Autodesk Fusion 360 part; units mm, degrees
(part 2 of 2)
  spline S19 degree 5 poles (10.4079, -1.3878) (10.4039, -1.3845) (10.3958, -1.3779) (10.3838, -1.3681) (10.3676, -1.3551) (10.3475, -1.3389) (10.3272, -1.3228) (10.3069, -1.3069) (10.2866, -1.2911) (10.2663, -1.2755) (10.2458, -1.2599) (10.2254, -1.2445) (10.2049, -1.2292) (10.1844, -1.214) (10.1638, -1.199) (10.1432, -1.1841) (10.1225, -1.1693) (10.1018, -1.1547) (10.0811, -1.1402) (10.0603, -1.1258) (10.0395, -1.1116) (10.0186, -1.0975) (9.9977, -1.0835) (9.9768, -1.0697) (9.9558, -1.056) (9.9348, -1.0424) (9.9137, -1.029) (9.8926, -1.0157) (9.8715, -1.0026) (9.8503, -0.9896) (9.8291, -0.9768) (9.8078, -0.9641) (9.7866, -0.9516) (9.7652, -0.9392) (9.7439, -0.9269) (9.7225, -0.9149) (9.7011, -0.9029) (9.6796, -0.8911) (9.6581, -0.8795) (9.6366, -0.8681) (9.615, -0.8568) (9.5934, -0.8456) (9.5717, -0.8347) (9.5501, -0.8239) (9.5283, -0.8132) (9.5066, -0.8028) (9.4848, -0.7925) (9.463, -0.7824) (9.4412, -0.7724) (9.4193, -0.7627) (9.3974, -0.7531) (9.3754, -0.7438) (9.3534, -0.7346) (9.3314, -0.7257) (9.3094, -0.7169) (9.2873, -0.7084) (9.2652, -0.7) (9.2431, -0.6918) (9.2209, -0.6839) (9.1987, -0.6761) (9.1764, -0.6686) (9.1542, -0.6615) (9.1318, -0.6547) (9.1095, -0.6482) (9.0871, -0.6419) (9.0646, -0.636) (9.0422, -0.6301) (9.0197, -0.6245) (8.9973, -0.619) (8.9748, -0.6141) (8.9522, -0.6098) (8.934, -0.6071) (8.9203, -0.6056) (8.9112, -0.6048) (8.9066, -0.6045) knots -1 -1 -1 -1 -1 -1 -0.98571429 -0.97142857 -0.95714286 -0.94285714 -0.92857143 -0.91428571 -0.9 -0.88571429 -0.87142857 -0.85714286 -0.84285714 -0.82857143 -0.81428571 -0.8 -0.78571429 -0.77142857 -0.75714286 -0.74285714 -0.72857143 -0.71428571 -0.7 -0.68571429 -0.67142857 -0.65714286 -0.64285714 -0.62857143 -0.61428571 -0.6 -0.58571429 -0.57142857 -0.55714286 -0.54285714 -0.52857143 -0.51428571 -0.5 -0.48571429 -0.47142857 -0.45714286 -0.44285714 -0.42857143 -0.41428571 -0.4 -0.38571429 -0.37142857 -0.35714286 -0.34285714 -0.32857143 -0.31428571 -0.3 -0.28571429 -0.27142857 -0.25714286 -0.24285714 -0.22857143 -0.21428571 -0.2 -0.18571429 -0.17142857 -0.15714286 -0.14285714 -0.12857143 -0.11428571 -0.1 -0.08571429 -0.07142857 -0.05714286 -0.04285714 -0.02857143 -0.01428571 0 0 0 0 0 0
  line L19 (8.9066, -0.6045) -> (8.2303, -0.5577)
  arc A20 (8.2303, -0.5577) -> (8.2303, 0.5577) centre (0, 0) ccw
  line L20 (8.2303, 0.5577) -> (8.9066, 0.6045)
  spline S20 degree 5 poles (8.9066, 0.6045) (8.9112, 0.6048) (8.9203, 0.6056) (8.934, 0.6071) (8.9522, 0.6098) (8.9748, 0.6141) (8.9973, 0.619) (9.0197, 0.6245) (9.0422, 0.6301) (9.0646, 0.636) (9.0871, 0.6419) (9.1095, 0.6482) (9.1318, 0.6547) (9.1542, 0.6615) (9.1764, 0.6686) (9.1987, 0.6761) (9.2209, 0.6839) (9.2431, 0.6918) (9.2652, 0.7) (9.2873, 0.7084) (9.3094, 0.7169) (9.3314, 0.7257) (9.3534, 0.7346) (9.3754, 0.7438) (9.3974, 0.7531) (9.4193, 0.7627) (9.4412, 0.7724) (9.463, 0.7824) (9.4848, 0.7925) (9.5066, 0.8028) (9.5283, 0.8132) (9.5501, 0.8239) (9.5717, 0.8347) (9.5934, 0.8456) (9.615, 0.8568) (9.6366, 0.8681) (9.6581, 0.8795) (9.6796, 0.8911) (9.7011, 0.9029) (9.7225, 0.9149) (9.7439, 0.9269) (9.7652, 0.9392) (9.7866, 0.9516) (9.8078, 0.9641) (9.8291, 0.9768) (9.8503, 0.9896) (9.8715, 1.0026) (9.8926, 1.0157) (9.9137, 1.029) (9.9348, 1.0424) (9.9558, 1.056) (9.9768, 1.0697) (9.9977, 1.0835) (10.0186, 1.0975) (10.0395, 1.1116) (10.0603, 1.1258) (10.0811, 1.1402) (10.1018, 1.1547) (10.1225, 1.1693) (10.1432, 1.1841) (10.1638, 1.199) (10.1844, 1.214) (10.2049, 1.2292) (10.2254, 1.2445) (10.2458, 1.2599) (10.2663, 1.2755) (10.2866, 1.2911) (10.3069, 1.3069) (10.3272, 1.3228) (10.3475, 1.3389) (10.3676, 1.3551) (10.3838, 1.3681) (10.3958, 1.3779) (10.4039, 1.3845) (10.4079, 1.3878) knots 0 0 0 0 0 0 0.01428571 0.02857143 0.04285714 0.05714286 0.07142857 0.08571429 0.1 0.11428571 0.12857143 0.14285714 0.15714286 0.17142857 0.18571429 0.2 0.21428571 0.22857143 0.24285714 0.25714286 0.27142857 0.28571429 0.3 0.31428571 0.32857143 0.34285714 0.35714286 0.37142857 0.38571429 0.4 0.41428571 0.42857143 0.44285714 0.45714286 0.47142857 0.48571429 0.5 0.51428571 0.52857143 0.54285714 0.55714286 0.57142857 0.58571429 0.6 0.61428571 0.62857143 0.64285714 0.65714286 0.67142857 0.68571429 0.7 0.71428571 0.72857143 0.74285714 0.75714286 0.77142857 0.78571429 0.8 0.81428571 0.82857143 0.84285714 0.85714286 0.87142857 0.88571429 0.9 0.91428571 0.92857143 0.94285714 0.95714286 0.97142857 0.98571429 1 1 1 1 1 1
  arc A21 (10.4079, 1.3878) -> (10.2946, 2.0668) centre (0, 0) ccw
  spline S21 degree 5 poles (10.2946, 2.0668) (10.2897, 2.0687) (10.28, 2.0723) (10.2654, 2.0776) (10.2459, 2.0847) (10.2215, 2.0935) (10.1972, 2.1021) (10.1728, 2.1105) (10.1485, 2.1189) (10.1241, 2.1271) (10.0998, 2.1352) (10.0754, 2.1431) (10.0511, 2.1509) (10.0267, 2.1586) (10.0024, 2.1661) (9.9781, 2.1735) (9.9537, 2.1808) (9.9294, 2.1879) (9.9051, 2.1949) (9.8807, 2.2018) (9.8564, 2.2085) (9.8321, 2.215) (9.8078, 2.2214) (9.7835, 2.2277) (9.7592, 2.2339) (9.7349, 2.2399) (9.7107, 2.2457) (9.6864, 2.2514) (9.6622, 2.257) (9.6379, 2.2624) (9.6137, 2.2676) (9.5895, 2.2727) (9.5653, 2.2777) (9.5411, 2.2825) (9.5169, 2.2871) (9.4927, 2.2916) (9.4686, 2.2959) (9.4445, 2.3001) (9.4204, 2.3041) (9.3963, 2.308) (9.3722, 2.3116) (9.3481, 2.3152) (9.3241, 2.3185) (9.3001, 2.3217) (9.2761, 2.3247) (9.2522, 2.3275) (9.2282, 2.3302) (9.2043, 2.3327) (9.1804, 2.335) (9.1566, 2.3371) (9.1327, 2.339) (9.1089, 2.3407) (9.0852, 2.3423) (9.0614, 2.3436) (9.0378, 2.3447) (9.0141, 2.3456) (8.9905, 2.3463) (8.9669, 2.3469) (8.9433, 2.3472) (8.9198, 2.3473) (8.8964, 2.3472) (8.873, 2.3467) (8.8496, 2.3459) (8.8264, 2.3448) (8.8031, 2.3434) (8.78, 2.3418) (8.7569, 2.34) (8.7338, 2.3381) (8.7108, 2.3359) (8.6879, 2.3333) (8.6651, 2.33) (8.6471, 2.3267) (8.6336, 2.3236) (8.6247, 2.3214) (8.6203, 2.3202) knots -1 -1 -1 -1 -1 -1 -0.98571429 -0.97142857 -0.95714286 -0.94285714 -0.92857143 -0.91428571 -0.9 -0.88571429 -0.87142857 -0.85714286 -0.84285714 -0.82857143 -0.81428571 -0.8 -0.78571429 -0.77142857 -0.75714286 -0.74285714 -0.72857143 -0.71428571 -0.7 -0.68571429 -0.67142857 -0.65714286 -0.64285714 -0.62857143 -0.61428571 -0.6 -0.58571429 -0.57142857 -0.55714286 -0.54285714 -0.52857143 -0.51428571 -0.5 -0.48571429 -0.47142857 -0.45714286 -0.44285714 -0.42857143 -0.41428571 -0.4 -0.38571429 -0.37142857 -0.35714286 -0.34285714 -0.32857143 -0.31428571 -0.3 -0.28571429 -0.27142857 -0.25714286 -0.24285714 -0.22857143 -0.21428571 -0.2 -0.18571429 -0.17142857 -0.15714286 -0.14285714 -0.12857143 -0.11428571 -0.1 -0.08571429 -0.07142857 -0.05714286 -0.04285714 -0.02857143 -0.01428571 0 0 0 0 0 0
  line L21 (8.6203, 2.3202) -> (7.9655, 2.1449)
  arc A22 (7.9655, 2.1449) -> (7.6033, 3.1998) centre (0, 0) ccw
  line L22 (7.6033, 3.1998) -> (8.2277, 3.4637)
  spline S22 degree 5 poles (8.2277, 3.4637) (8.2319, 3.4655) (8.2404, 3.4692) (8.2528, 3.4751) (8.2691, 3.4835) (8.2891, 3.4949) (8.3088, 3.5069) (8.3283, 3.5193) (8.3477, 3.532) (8.367, 3.5448) (8.3863, 3.5577) (8.4054, 3.5709) (8.4245, 3.5843) (8.4434, 3.598) (8.4621, 3.612) (8.4807, 3.6263) (8.4992, 3.6408) (8.5176, 3.6556) (8.5359, 3.6705) (8.5541, 3.6856) (8.5722, 3.7008) (8.5902, 3.7162) (8.6081, 3.7319) (8.6259, 3.7476) (8.6437, 3.7636) (8.6613, 3.7798) (8.6788, 3.7961) (8.6962, 3.8126) (8.7136, 3.8293) (8.7308, 3.8461) (8.748, 3.863) (8.7651, 3.8801) (8.7821, 3.8974) (8.799, 3.9148) (8.8158, 3.9323) (8.8326, 3.95) (8.8492, 3.9678) (8.8658, 3.9858) (8.8822, 4.0039) (8.8986, 4.0222) (8.9149, 4.0405) (8.9312, 4.0591) (8.9473, 4.0777) (8.9634, 4.0965) (8.9794, 4.1154) (8.9952, 4.1344) (9.0111, 4.1536) (9.0268, 4.1728) (9.0424, 4.1922) (9.058, 4.2118) (9.0735, 4.2314) (9.0889, 4.2512) (9.1042, 4.271) (9.1194, 4.291) (9.1346, 4.3112) (9.1496, 4.3314) (9.1646, 4.3517) (9.1795, 4.3722) (9.1944, 4.3928) (9.2091, 4.4134) (9.2238, 4.4342) (9.2383, 4.4551) (9.2528, 4.4761) (9.2673, 4.4972) (9.2816, 4.5185) (9.2959, 4.5398) (9.31, 4.5612) (9.3241, 4.5828) (9.3381, 4.6044) (9.3521, 4.6262) (9.3659, 4.648) (9.3769, 4.6656) (9.3851, 4.6788) (9.3906, 4.6876) (9.3933, 4.692) knots 0 0 0 0 0 0 0.01428571 0.02857143 0.04285714 0.05714286 0.07142857 0.08571429 0.1 0.11428571 0.12857143 0.14285714 0.15714286 0.17142857 0.18571429 0.2 0.21428571 0.22857143 0.24285714 0.25714286 0.27142857 0.28571429 0.3 0.31428571 0.32857143 0.34285714 0.35714286 0.37142857 0.38571429 0.4 0.41428571 0.42857143 0.44285714 0.45714286 0.47142857 0.48571429 0.5 0.51428571 0.52857143 0.54285714 0.55714286 0.57142857 0.58571429 0.6 0.61428571 0.62857143 0.64285714 0.65714286 0.67142857 0.68571429 0.7 0.71428571 0.72857143 0.74285714 0.75714286 0.77142857 0.78571429 0.8 0.81428571 0.82857143 0.84285714 0.85714286 0.87142857 0.88571429 0.9 0.91428571 0.92857143 0.94285714 0.95714286 0.97142857 0.98571429 1 1 1 1 1 1
  arc A23 (9.3933, 4.692) -> (9.0657, 5.2975) centre (0, 0) ccw
  spline S23 degree 5 poles (9.0657, 5.2975) (9.0605, 5.2976) (9.0501, 5.2979) (9.0345, 5.2982) (9.0138, 5.2986) (8.988, 5.299) (8.9621, 5.2992) (8.9364, 5.2993) (8.9106, 5.2993) (8.8849, 5.2991) (8.8593, 5.2989) (8.8337, 5.2985) (8.8081, 5.298) (8.7826, 5.2973) (8.7571, 5.2965) (8.7317, 5.2956) (8.7063, 5.2946) (8.681, 5.2934) (8.6557, 5.2921) (8.6305, 5.2907) (8.6053, 5.2892) (8.5802, 5.2875) (8.5551, 5.2857) (8.5301, 5.2837) (8.5051, 5.2816) (8.4802, 5.2794) (8.4553, 5.2771) (8.4305, 5.2746) (8.4058, 5.272) (8.3811, 5.2692) (8.3565, 5.2663) (8.3319, 5.2633) (8.3074, 5.2601) (8.283, 5.2568) (8.2586, 5.2533) (8.2343, 5.2497) (8.2101, 5.246) (8.1859, 5.2421) (8.1618, 5.2381) (8.1378, 5.2339) (8.1138, 5.2295) (8.0899, 5.2251) (8.0661, 5.2204) (8.0424, 5.2156) (8.0187, 5.2107) (7.9951, 5.2056) (7.9716, 5.2003) (7.9482, 5.1949) (7.9248, 5.1893) (7.9016, 5.1836) (7.8784, 5.1777) (7.8554, 5.1716) (7.8324, 5.1653) (7.8095, 5.1588) (7.7867, 5.1522) (7.7641, 5.1454) (7.7415, 5.1384) (7.719, 5.1312) (7.6966, 5.1239) (7.6743, 5.1164) (7.6522, 5.1086) (7.6302, 5.1006) (7.6084, 5.0923) (7.5868, 5.0837) (7.5653, 5.0748) (7.5439, 5.0658) (7.5226, 5.0566) (7.5014, 5.0473) (7.4803, 5.0377) (7.4595, 5.0278) (7.439, 5.0173) (7.4231, 5.0083) (7.4113, 5.0011) (7.4037, 4.9961) (7.3999, 4.9935) knots -1 -1 -1 -1 -1 -1 -0.98571429 -0.97142857 -0.95714286 -0.94285714 -0.92857143 -0.91428571 -0.9 -0.88571429 -0.87142857 -0.85714286 -0.84285714 -0.82857143 -0.81428571 -0.8 -0.78571429 -0.77142857 -0.75714286 -0.74285714 -0.72857143 -0.71428571 -0.7 -0.68571429 -0.67142857 -0.65714286 -0.64285714 -0.62857143 -0.61428571 -0.6 -0.58571429 -0.57142857 -0.55714286 -0.54285714 -0.52857143 -0.51428571 -0.5 -0.48571429 -0.47142857 -0.45714286 -0.44285714 -0.42857143 -0.41428571 -0.4 -0.38571429 -0.37142857 -0.35714286 -0.34285714 -0.32857143 -0.31428571 -0.3 -0.28571429 -0.27142857 -0.25714286 -0.24285714 -0.22857143 -0.21428571 -0.2 -0.18571429 -0.17142857 -0.15714286 -0.14285714 -0.12857143 -0.11428571 -0.1 -0.08571429 -0.07142857 -0.05714286 -0.04285714 -0.02857143 -0.01428571 0 0 0 0 0 0
  line L23 (7.3999, 4.9935) -> (6.8374, 4.6151)
  arc A24 (6.8374, 4.6151) -> (6.1524, 5.4952) centre (0, 0) ccw
  line L24 (6.1524, 5.4952) -> (6.6572, 5.9476)
  spline S24 degree 5 poles (6.6572, 5.9476) (6.6607, 5.9507) (6.6674, 5.9569) (6.6773, 5.9665) (6.69, 5.9797) (6.7052, 5.997) (6.7199, 6.0147) (6.7343, 6.0328) (6.7485, 6.0511) (6.7627, 6.0695) (6.7767, 6.088) (6.7905, 6.1066) (6.8042, 6.1255) (6.8176, 6.1446) (6.8308, 6.1639) (6.8438, 6.1835) (6.8565, 6.2033) (6.8691, 6.2232) (6.8816, 6.2432) (6.8939, 6.2634) (6.9061, 6.2837) (6.9181, 6.3041) (6.93, 6.3247) (6.9417, 6.3454) (6.9533, 6.3663) (6.9647, 6.3873) (6.976, 6.4084) (6.9871, 6.4297) (6.9981, 6.4511) (7.009, 6.4726) (7.0197, 6.4942) (7.0303, 6.5159) (7.0408, 6.5377) (7.0511, 6.5597) (7.0613, 6.5817) (7.0714, 6.6039) (7.0814, 6.6262) (7.0912, 6.6486) (7.1009, 6.671) (7.1105, 6.6936) (7.12, 6.7163) (7.1293, 6.7391) (7.1385, 6.7619) (7.1476, 6.7849) (7.1566, 6.808) (7.1654, 6.8311) (7.1742, 6.8544) (7.1828, 6.8777) (7.1913, 6.9012) (7.1996, 6.9247) (7.2079, 6.9483) (7.2161, 6.972) (7.2241, 6.9957) (7.232, 7.0196) (7.2398, 7.0436) (7.2475, 7.0676) (7.2551, 7.0917) (7.2625, 7.1159) (7.2699, 7.1401) (7.2771, 7.1645) (7.2842, 7.1889) (7.2912, 7.2134) (7.2981, 7.238) (7.3049, 7.2626) (7.3116, 7.2874) (7.3181, 7.3122) (7.3246, 7.3371) (7.3309, 7.362) (7.3371, 7.387) (7.3432, 7.4121) (7.3492, 7.4373) (7.354, 7.4575) (7.3574, 7.4726) (7.3597, 7.4827) (7.3609, 7.4878) knots 0 0 0 0 0 0 0.01428571 0.02857143 0.04285714 0.05714286 0.07142857 0.08571429 0.1 0.11428571 0.12857143 0.14285714 0.15714286 0.17142857 0.18571429 0.2 0.21428571 0.22857143 0.24285714 0.25714286 0.27142857 0.28571429 0.3 0.31428571 0.32857143 0.34285714 0.35714286 0.37142857 0.38571429 0.4 0.41428571 0.42857143 0.44285714 0.45714286 0.47142857 0.48571429 0.5 0.51428571 0.52857143 0.54285714 0.55714286 0.57142857 0.58571429 0.6 0.61428571 0.62857143 0.64285714 0.65714286 0.67142857 0.68571429 0.7 0.71428571 0.72857143 0.74285714 0.75714286 0.77142857 0.78571429 0.8 0.81428571 0.82857143 0.84285714 0.85714286 0.87142857 0.88571429 0.9 0.91428571 0.92857143 0.94285714 0.95714286 0.97142857 0.98571429 1 1 1 1 1 1
  arc A25 (7.3609, 7.4878) -> (6.8544, 7.9541) centre (0, 0) ccw
  spline S25 degree 5 poles (6.8544, 7.9541) (6.8494, 7.9525) (6.8395, 7.9494) (6.8247, 7.9447) (6.805, 7.9383) (6.7804, 7.9302) (6.7559, 7.9221) (6.7315, 7.9138) (6.7071, 7.9054) (6.6829, 7.897) (6.6587, 7.8884) (6.6346, 7.8797) (6.6106, 7.8709) (6.5867, 7.862) (6.5628, 7.853) (6.5391, 7.8439) (6.5154, 7.8347) (6.4918, 7.8253) (6.4683, 7.8159) (6.4449, 7.8064) (6.4216, 7.7967) (6.3984, 7.787) (6.3753, 7.7771) (6.3523, 7.7671) (6.3293, 7.7571) (6.3065, 7.7469) (6.2837, 7.7366) (6.2611, 7.7262) (6.2385, 7.7157) (6.2161, 7.7051) (6.1937, 7.6943) (6.1715, 7.6835) (6.1494, 7.6725) (6.1273, 7.6614) (6.1054, 7.6503) (6.0836, 7.639) (6.0619, 7.6275) (6.0403, 7.616) (6.0188, 7.6044) (5.9974, 7.5926) (5.9761, 7.5807) (5.955, 7.5687) (5.934, 7.5566) (5.9131, 7.5444) (5.8923, 7.532) (5.8717, 7.5195) (5.8511, 7.5069) (5.8307, 7.4942) (5.8105, 7.4813) (5.7903, 7.4684) (5.7704, 7.4553) (5.7505, 7.442) (5.7308, 7.4286) (5.7113, 7.4151) (5.6919, 7.4014) (5.6727, 7.3876) (5.6536, 7.3736) (5.6347, 7.3596) (5.6159, 7.3454) (5.5972, 7.331) (5.5788, 7.3165) (5.5606, 7.3018) (5.5427, 7.2868) (5.525, 7.2716) (5.5076, 7.2563) (5.4903, 7.2408) (5.4731, 7.2252) (5.4561, 7.2095) (5.4393, 7.1936) (5.4228, 7.1775) (5.4068, 7.1609) (5.3947, 7.1472) (5.3859, 7.1366) (5.3803, 7.1293) (5.3775, 7.1257) knots -1 -1 -1 -1 -1 -1 -0.98571429 -0.97142857 -0.95714286 -0.94285714 -0.92857143 -0.91428571 -0.9 -0.88571429 -0.87142857 -0.85714286 -0.84285714 -0.82857143 -0.81428571 -0.8 -0.78571429 -0.77142857 -0.75714286 -0.74285714 -0.72857143 -0.71428571 -0.7 -0.68571429 -0.67142857 -0.65714286 -0.64285714 -0.62857143 -0.61428571 -0.6 -0.58571429 -0.57142857 -0.55714286 -0.54285714 -0.52857143 -0.51428571 -0.5 -0.48571429 -0.47142857 -0.45714286 -0.44285714 -0.42857143 -0.41428571 -0.4 -0.38571429 -0.37142857 -0.35714286 -0.34285714 -0.32857143 -0.31428571 -0.3 -0.28571429 -0.27142857 -0.25714286 -0.24285714 -0.22857143 -0.21428571 -0.2 -0.18571429 -0.17142857 -0.15714286 -0.14285714 -0.12857143 -0.11428571 -0.1 -0.08571429 -0.07142857 -0.05714286 -0.04285714 -0.02857143 -0.01428571 0 0 0 0 0 0
  line L25 (5.3775, 7.1257) -> (4.9684, 6.5851)
  arc A26 (4.9684, 6.5851) -> (4.0347, 7.1952) centre (0, 0) ccw
  line L26 (4.0347, 7.1952) -> (4.3654, 7.7869)
  spline S26 degree 5 poles (4.3654, 7.7869) (4.3676, 7.7909) (4.372, 7.799) (4.3782, 7.8113) (4.3859, 7.828) (4.3947, 7.8492) (4.4028, 7.8708) (4.4106, 7.8926) (4.4181, 7.9145) (4.4255, 7.9364) (4.4327, 7.9585) (4.4398, 7.9807) (4.4466, 8.0029) (4.4531, 8.0254) (4.4593, 8.0479) (4.4652, 8.0706) (4.4708, 8.0935) (4.4763, 8.1164) (4.4816, 8.1394) (4.4866, 8.1625) (4.4916, 8.1856) (4.4963, 8.2089) (4.5009, 8.2322) (4.5052, 8.2556) (4.5094, 8.2791) (4.5134, 8.3027) (4.5172, 8.3263) (4.5208, 8.35) (4.5243, 8.3738) (4.5276, 8.3977) (4.5307, 8.4216) (4.5337, 8.4456) (4.5365, 8.4696) (4.5392, 8.4938) (4.5417, 8.5179) (4.544, 8.5422) (4.5462, 8.5665) (4.5482, 8.5908) (4.5501, 8.6152) (4.5518, 8.6397) (4.5534, 8.6642) (4.5548, 8.6888) (4.5561, 8.7134) (4.5573, 8.7381) (4.5583, 8.7628) (4.5591, 8.7876) (4.5598, 8.8124) (4.5604, 8.8373) (4.5608, 8.8622) (4.5611, 8.8872) (4.5613, 8.9122) (4.5613, 8.9373) (4.5611, 8.9624) (4.5609, 8.9875) (4.5605, 9.0127) (4.56, 9.0379) (4.5593, 9.0632) (4.5585, 9.0885) (4.5576, 9.1138) (4.5565, 9.1392) (4.5553, 9.1646) (4.554, 9.19) (4.5525, 9.2155) (4.5509, 9.241) (4.5492, 9.2666) (4.5473, 9.2922) (4.5454, 9.3178) (4.5432, 9.3434) (4.541, 9.3691) (4.5386, 9.3948) (4.5362, 9.4206) (4.5341, 9.4412) (4.5324, 9.4567) (4.5313, 9.467) (4.5308, 9.4722) knots 0 0 0 0 0 0 0.01428571 0.02857143 0.04285714 0.05714286 0.07142857 0.08571429 0.1 0.11428571 0.12857143 0.14285714 0.15714286 0.17142857 0.18571429 0.2 0.21428571 0.22857143 0.24285714 0.25714286 0.27142857 0.28571429 0.3 0.31428571 0.32857143 0.34285714 0.35714286 0.37142857 0.38571429 0.4 0.41428571 0.42857143 0.44285714 0.45714286 0.47142857 0.48571429 0.5 0.51428571 0.52857143 0.54285714 0.55714286 0.57142857 0.58571429 0.6 0.61428571 0.62857143 0.64285714 0.65714286 0.67142857 0.68571429 0.7 0.71428571 0.72857143 0.74285714 0.75714286 0.77142857 0.78571429 0.8 0.81428571 0.82857143 0.84285714 0.85714286 0.87142857 0.88571429 0.9 0.91428571 0.92857143 0.94285714 0.95714286 0.97142857 0.98571429 1 1 1 1 1 1
  arc A27 (4.5308, 9.4722) -> (3.9003, 9.7487) centre (0, 0) ccw
  spline S27 degree 5 poles (3.9003, 9.7487) (3.8961, 9.7456) (3.8878, 9.7395) (3.8753, 9.7302) (3.8587, 9.7178) (3.8381, 9.7021) (3.8175, 9.6865) (3.7971, 9.6707) (3.7768, 9.6549) (3.7566, 9.639) (3.7366, 9.623) (3.7166, 9.607) (3.6967, 9.5909) (3.677, 9.5747) (3.6574, 9.5584) (3.6379, 9.5421) (3.6185, 9.5257) (3.5992, 9.5092) (3.5801, 9.4927) (3.561, 9.4761) (3.5421, 9.4594) (3.5233, 9.4426) (3.5046, 9.4258) (3.4861, 9.4089) (3.4677, 9.3919) (3.4494, 9.3749) (3.4312, 9.3577) (3.4132, 9.3405) (3.3952, 9.3233) (3.3775, 9.3059) (3.3598, 9.2885) (3.3423, 9.271) (3.3249, 9.2535) (3.3077, 9.2359) (3.2906, 9.2182) (3.2736, 9.2004) (3.2568, 9.1826) (3.2401, 9.1646) (3.2235, 9.1466) (3.2071, 9.1286) (3.1909, 9.1104) (3.1748, 9.0922) (3.1588, 9.0739) (3.143, 9.0556) (3.1274, 9.0371) (3.1119, 9.0186) (3.0966, 9) (3.0815, 8.9814) (3.0665, 8.9626) (3.0516, 8.9438) (3.037, 8.9249) (3.0225, 8.906) (3.0083, 8.8869) (2.9942, 8.8678) (2.9803, 8.8485) (2.9666, 8.8292) (2.9531, 8.8098) (2.9397, 8.7904) (2.9265, 8.7708) (2.9136, 8.7512) (2.9009, 8.7315) (2.8885, 8.7117) (2.8764, 8.6917) (2.8646, 8.6716) (2.853, 8.6514) (2.8417, 8.6311) (2.8306, 8.6108) (2.8196, 8.5904) (2.8088, 8.57) (2.7984, 8.5494) (2.7887, 8.5285) (2.7817, 8.5116) (2.7769, 8.4987) (2.7739, 8.49) (2.7725, 8.4856) knots -1 -1 -1 -1 -1 -1 -0.98571429 -0.97142857 -0.95714286 -0.94285714 -0.92857143 -0.91428571 -0.9 -0.88571429 -0.87142857 -0.85714286 -0.84285714 -0.82857143 -0.81428571 -0.8 -0.78571429 -0.77142857 -0.75714286 -0.74285714 -0.72857143 -0.71428571 -0.7 -0.68571429 -0.67142857 -0.65714286 -0.64285714 -0.62857143 -0.61428571 -0.6 -0.58571429 -0.57142857 -0.55714286 -0.54285714 -0.52857143 -0.51428571 -0.5 -0.48571429 -0.47142857 -0.45714286 -0.44285714 -0.42857143 -0.41428571 -0.4 -0.38571429 -0.37142857 -0.35714286 -0.34285714 -0.32857143 -0.31428571 -0.3 -0.28571429 -0.27142857 -0.25714286 -0.24285714 -0.22857143 -0.21428571 -0.2 -0.18571429 -0.17142857 -0.15714286 -0.14285714 -0.12857143 -0.11428571 -0.1 -0.08571429 -0.07142857 -0.05714286 -0.04285714 -0.02857143 -0.01428571 0 0 0 0 0 0
  line L27 (2.7725, 8.4856) -> (2.561, 7.8416)
  arc A28 (2.561, 7.8416) -> (1.4798, 8.1154) centre (0, 0) ccw
  line L28 (1.4798, 8.1154) -> (1.6004, 8.7824)
  spline S28 degree 5 poles (1.6004, 8.7824) (1.6012, 8.787) (1.6028, 8.796) (1.6047, 8.8097) (1.6065, 8.8279) (1.6079, 8.8509) (1.6086, 8.8739) (1.6089, 8.897) (1.6089, 8.9202) (1.6087, 8.9434) (1.6084, 8.9666) (1.6079, 8.9898) (1.6071, 9.0131) (1.606, 9.0364) (1.6045, 9.0598) (1.6027, 9.0832) (1.6007, 9.1066) (1.5984, 9.1301) (1.5959, 9.1535) (1.5932, 9.177) (1.5903, 9.2005) (1.5873, 9.224) (1.584, 9.2476) (1.5805, 9.2711) (1.5769, 9.2947) (1.573, 9.3183) (1.5689, 9.3419) (1.5646, 9.3655) (1.5602, 9.3891) (1.5555, 9.4128) (1.5507, 9.4364) (1.5458, 9.4601) (1.5406, 9.4837) (1.5353, 9.5074) (1.5298, 9.5311) (1.5241, 9.5548) (1.5183, 9.5785) (1.5123, 9.6022) (1.5062, 9.6259) (1.4999, 9.6496) (1.4934, 9.6733) (1.4868, 9.697) (1.48, 9.7207) (1.4731, 9.7444) (1.466, 9.7681) (1.4587, 9.7918) (1.4514, 9.8155) (1.4438, 9.8392) (1.4361, 9.8629) (1.4283, 9.8867) (1.4203, 9.9104) (1.4122, 9.9341) (1.4039, 9.9578) (1.3955, 9.9814) (1.387, 10.0051) (1.3783, 10.0288) (1.3695, 10.0525) (1.3605, 10.0762) (1.3514, 10.0998) (1.3421, 10.1235) (1.3327, 10.1471) (1.3232, 10.1708) (1.3136, 10.1944) (1.3038, 10.218) (1.2938, 10.2416) (1.2838, 10.2652) (1.2736, 10.2888) (1.2633, 10.3124) (1.2528, 10.3359) (1.2422, 10.3595) (1.2315, 10.383) (1.2228, 10.4019) (1.2163, 10.416) (1.2119, 10.4254) (1.2097, 10.4301) knots 0 0 0 0 0 0 0.01428571 0.02857143 0.04285714 0.05714286 0.07142857 0.08571429 0.1 0.11428571 0.12857143 0.14285714 0.15714286 0.17142857 0.18571429 0.2 0.21428571 0.22857143 0.24285714 0.25714286 0.27142857 0.28571429 0.3 0.31428571 0.32857143 0.34285714 0.35714286 0.37142857 0.38571429 0.4 0.41428571 0.42857143 0.44285714 0.45714286 0.47142857 0.48571429 0.5 0.51428571 0.52857143 0.54285714 0.55714286 0.57142857 0.58571429 0.6 0.61428571 0.62857143 0.64285714 0.65714286 0.67142857 0.68571429 0.7 0.71428571 0.72857143 0.74285714 0.75714286 0.77142857 0.78571429 0.8 0.81428571 0.82857143 0.84285714 0.85714286 0.87142857 0.88571429 0.9 0.91428571 0.92857143 0.94285714 0.95714286 0.97142857 0.98571429 1 1 1 1 1 1
  arc A29 (1.2097, 10.4301) -> (0.5236, 10.4869) centre (0, 0) ccw
  spline S29 degree 5 poles (0.5236, 10.4869) (0.5206, 10.4827) (0.5147, 10.4741) (0.5059, 10.4613) (0.4943, 10.4441) (0.4798, 10.4227) (0.4655, 10.4012) (0.4513, 10.3797) (0.4373, 10.3581) (0.4233, 10.3365) (0.4095, 10.3149) (0.3958, 10.2932) (0.3823, 10.2716) (0.3689, 10.2498) (0.3556, 10.2281) (0.3424, 10.2063) (0.3294, 10.1845) (0.3166, 10.1627) (0.3038, 10.1408) (0.2912, 10.1189) (0.2787, 10.097) (0.2664, 10.075) (0.2542, 10.053) (0.2421, 10.031) (0.2302, 10.009) (0.2185, 9.9869) (0.2068, 9.9648) (0.1954, 9.9427) (0.184, 9.9205) (0.1728, 9.8984) (0.1618, 9.8762) (0.1509, 9.854) (0.1402, 9.8317) (0.1296, 9.8094) (0.1191, 9.7871) (0.1089, 9.7648) (0.0987, 9.7425) (0.0888, 9.7201) (0.079, 9.6977) (0.0693, 9.6753) (0.0598, 9.6529) (0.0505, 9.6304) (0.0414, 9.608) (0.0324, 9.5855) (0.0236, 9.563) (0.015, 9.5404) (0.0065, 9.5179) (-0.0018, 9.4953) (-0.0099, 9.4727) (-0.0178, 9.4501) (-0.0255, 9.4275) (-0.033, 9.4048) (-0.0403, 9.3822) (-0.0474, 9.3595) (-0.0543, 9.3368) (-0.061, 9.3141) (-0.0675, 9.2914) (-0.0738, 9.2686) (-0.0799, 9.2459) (-0.0858, 9.2231) (-0.0914, 9.2003) (-0.0967, 9.1775) (-0.1017, 9.1547) (-0.1063, 9.1319) (-0.1106, 9.109) (-0.1148, 9.0862) (-0.1187, 9.0633) (-0.1225, 9.0405) (-0.1261, 9.0177) (-0.1292, 8.9948) (-0.1316, 8.9719) (-0.1328, 8.9536) (-0.1331, 8.9399) (-0.1331, 8.9307) (-0.133, 8.9261) knots -1 -1 -1 -1 -1 -1 -0.98571429 -0.97142857 -0.95714286 -0.94285714 -0.92857143 -0.91428571 -0.9 -0.88571429 -0.87142857 -0.85714286 -0.84285714 -0.82857143 -0.81428571 -0.8 -0.78571429 -0.77142857 -0.75714286 -0.74285714 -0.72857143 -0.71428571 -0.7 -0.68571429 -0.67142857 -0.65714286 -0.64285714 -0.62857143 -0.61428571 -0.6 -0.58571429 -0.57142857 -0.55714286 -0.54285714 -0.52857143 -0.51428571 -0.5 -0.48571429 -0.47142857 -0.45714286 -0.44285714 -0.42857143 -0.41428571 -0.4 -0.38571429 -0.37142857 -0.35714286 -0.34285714 -0.32857143 -0.31428571 -0.3 -0.28571429 -0.27142857 -0.25714286 -0.24285714 -0.22857143 -0.21428571 -0.2 -0.18571429 -0.17142857 -0.15714286 -0.14285714 -0.12857143 -0.11428571 -0.1 -0.08571429 -0.07142857 -0.05714286 -0.04285714 -0.02857143 -0.01428571 0 0 0 0 0 0
  line L29 (-0.133, 8.9261) -> (-0.1239, 8.2483)
  arc A30 (-0.1239, 8.2483) -> (-1.2354, 8.1562) centre (0, 0) ccw
  line L30 (-1.2354, 8.1562) -> (-1.338, 8.8262)
  spline S30 degree 5 poles (-1.338, 8.8262) (-1.3386, 8.8308) (-1.3402, 8.8398) (-1.3428, 8.8534) (-1.3469, 8.8712) (-1.3531, 8.8934) (-1.3599, 8.9154) (-1.3672, 8.9374) (-1.3747, 8.9593) (-1.3823, 8.9812) (-1.3902, 9.003) (-1.3982, 9.0248) (-1.4065, 9.0466) (-1.4152, 9.0683) (-1.4241, 9.0899) (-1.4334, 9.1114) (-1.443, 9.1329) (-1.4528, 9.1544) (-1.4627, 9.1757) (-1.4729, 9.1971) (-1.4832, 9.2184) (-1.4938, 9.2396) (-1.5045, 9.2608) (-1.5154, 9.282) (-1.5266, 9.3031) (-1.5379, 9.3241) (-1.5494, 9.3451) (-1.5611, 9.3661) (-1.573, 9.387) (-1.5851, 9.4078) (-1.5973, 9.4286) (-1.6097, 9.4494) (-1.6222, 9.4701) (-1.6349, 9.4908) (-1.6478, 9.5114) (-1.6609, 9.532) (-1.6741, 9.5525) (-1.6874, 9.5729) (-1.7009, 9.5934) (-1.7146, 9.6137) (-1.7284, 9.6341) (-1.7424, 9.6543) (-1.7565, 9.6745) (-1.7707, 9.6947) (-1.7851, 9.7149) (-1.7997, 9.7349) (-1.8144, 9.755) (-1.8292, 9.7749) (-1.8442, 9.7949) (-1.8593, 9.8147) (-1.8745, 9.8346) (-1.8899, 9.8543) (-1.9054, 9.8741) (-1.9211, 9.8938) (-1.9368, 9.9134) (-1.9527, 9.933) (-1.9688, 9.9525) (-1.985, 9.9719) (-2.0013, 9.9914) (-2.0177, 10.0107) (-2.0342, 10.0301) (-2.0509, 10.0493) (-2.0677, 10.0685) (-2.0847, 10.0877) (-2.1017, 10.1068) (-2.1189, 10.1259) (-2.1362, 10.1449) (-2.1536, 10.1638) (-2.1711, 10.1827) (-2.1888, 10.2015) (-2.2066, 10.2203) (-2.2209, 10.2353) (-2.2317, 10.2465) (-2.2389, 10.254) (-2.2425, 10.2577) knots 0 0 0 0 0 0 0.01428571 0.02857143 0.04285714 0.05714286 0.07142857 0.08571429 0.1 0.11428571 0.12857143 0.14285714 0.15714286 0.17142857 0.18571429 0.2 0.21428571 0.22857143 0.24285714 0.25714286 0.27142857 0.28571429 0.3 0.31428571 0.32857143 0.34285714 0.35714286 0.37142857 0.38571429 0.4 0.41428571 0.42857143 0.44285714 0.45714286 0.47142857 0.48571429 0.5 0.51428571 0.52857143 0.54285714 0.55714286 0.57142857 0.58571429 0.6 0.61428571 0.62857143 0.64285714 0.65714286 0.67142857 0.68571429 0.7 0.71428571 0.72857143 0.74285714 0.75714286 0.77142857 0.78571429 0.8 0.81428571 0.82857143 0.84285714 0.85714286 0.87142857 0.88571429 0.9 0.91428571 0.92857143 0.94285714 0.95714286 0.97142857 0.98571429 1 1 1 1 1 1
  arc A31 (-2.2425, 10.2577) -> (-2.9099, 10.0887) centre (0, 0) ccw
  spline S31 degree 5 poles (-2.9099, 10.0887) (-2.9113, 10.0837) (-2.9141, 10.0737) (-2.9183, 10.0587) (-2.9237, 10.0387) (-2.9304, 10.0137) (-2.937, 9.9888) (-2.9434, 9.9638) (-2.9497, 9.9389) (-2.9559, 9.9139) (-2.9619, 9.889) (-2.9678, 9.8641) (-2.9736, 9.8391) (-2.9792, 9.8142) (-2.9847, 9.7894) (-2.9901, 9.7645) (-2.9953, 9.7396) (-3.0004, 9.7148) (-3.0054, 9.69) (-3.0102, 9.6652) (-3.0149, 9.6404) (-3.0194, 9.6156) (-3.0238, 9.5909) (-3.028, 9.5661) (-3.0321, 9.5414) (-3.0361, 9.5167) (-3.0399, 9.4921) (-3.0436, 9.4674) (-3.0471, 9.4428) (-3.0505, 9.4182) (-3.0538, 9.3936) (-3.0569, 9.369) (-3.0598, 9.3445) (-3.0626, 9.32) (-3.0652, 9.2955) (-3.0677, 9.2711) (-3.07, 9.2467) (-3.0722, 9.2223) (-3.0742, 9.1979) (-3.076, 9.1736) (-3.0777, 9.1493) (-3.0792, 9.125) (-3.0806, 9.1008) (-3.0818, 9.0766) (-3.0828, 9.0525) (-3.0836, 9.0284) (-3.0843, 9.0043) (-3.0848, 8.9802) (-3.0851, 8.9562) (-3.0852, 8.9323) (-3.0852, 8.9084) (-3.085, 8.8845) (-3.0845, 8.8607) (-3.0839, 8.837) (-3.083, 8.8133) (-3.082, 8.7896) (-3.0807, 8.766) (-3.0793, 8.7425) (-3.0777, 8.7189) (-3.0759, 8.6955) (-3.0738, 8.6721) (-3.0714, 8.6489) (-3.0687, 8.6257) (-3.0657, 8.6026) (-3.0624, 8.5796) (-3.0588, 8.5566) (-3.0552, 8.5337) (-3.0513, 8.5109) (-3.0473, 8.4881) (-3.0428, 8.4655) (-3.0376, 8.4431) (-3.0328, 8.4254) (-3.0287, 8.4123) (-3.0257, 8.4036) (-3.0241, 8.3992) knots -1 -1 -1 -1 -1 -1 -0.98571429 -0.97142857 -0.95714286 -0.94285714 -0.92857143 -0.91428571 -0.9 -0.88571429 -0.87142857 -0.85714286 -0.84285714 -0.82857143 -0.81428571 -0.8 -0.78571429 -0.77142857 -0.75714286 -0.74285714 -0.72857143 -0.71428571 -0.7 -0.68571429 -0.67142857 -0.65714286 -0.64285714 -0.62857143 -0.61428571 -0.6 -0.58571429 -0.57142857 -0.55714286 -0.54285714 -0.52857143 -0.51428571 -0.5 -0.48571429 -0.47142857 -0.45714286 -0.44285714 -0.42857143 -0.41428571 -0.4 -0.38571429 -0.37142857 -0.35714286 -0.34285714 -0.32857143 -0.31428571 -0.3 -0.28571429 -0.27142857 -0.25714286 -0.24285714 -0.22857143 -0.21428571 -0.2 -0.18571429 -0.17142857 -0.15714286 -0.14285714 -0.12857143 -0.11428571 -0.1 -0.08571429 -0.07142857 -0.05714286 -0.04285714 -0.02857143 -0.01428571 0 0 0 0 0 0
  line L31 (-3.0241, 8.3992) -> (-2.7954, 7.7611)
  arc A32 (-2.7954, 7.7611) -> (-3.8168, 7.3131) centre (0, 0) ccw
  line L32 (-3.8168, 7.3131) -> (-4.1313, 7.9136)
  spline S32 degree 5 poles (-4.1313, 7.9136) (-4.1335, 7.9177) (-4.1378, 7.9257) (-4.1447, 7.9377) (-4.1544, 7.9532) (-4.1675, 7.9722) (-4.1811, 7.9908) (-4.1951, 8.0092) (-4.2093, 8.0275) (-4.2236, 8.0457) (-4.2381, 8.0638) (-4.2528, 8.0818) (-4.2677, 8.0997) (-4.283, 8.1174) (-4.2985, 8.135) (-4.3142, 8.1523) (-4.3303, 8.1695) (-4.3465, 8.1866) (-4.3628, 8.2036) (-4.3794, 8.2205) (-4.3961, 8.2373) (-4.4129, 8.254) (-4.43, 8.2706) (-4.4472, 8.287) (-4.4646, 8.3033) (-4.4821, 8.3196) (-4.4998, 8.3357) (-4.5177, 8.3517) (-4.5357, 8.3676) (-4.5539, 8.3834) (-4.5722, 8.3991) (-4.5907, 8.4147) (-4.6093, 8.4303) (-4.628, 8.4457) (-4.6469, 8.461) (-4.6659, 8.4762) (-4.685, 8.4913) (-4.7043, 8.5063) (-4.7237, 8.5213) (-4.7433, 8.5361) (-4.7629, 8.5508) (-4.7827, 8.5655) (-4.8026, 8.58) (-4.8227, 8.5945) (-4.8428, 8.6088) (-4.8631, 8.6231) (-4.8835, 8.6373) (-4.904, 8.6514) (-4.9246, 8.6653) (-4.9454, 8.6792) (-4.9662, 8.693) (-4.9872, 8.7068) (-5.0083, 8.7204) (-5.0295, 8.7339) (-5.0508, 8.7474) (-5.0722, 8.7607) (-5.0937, 8.774) (-5.1153, 8.7871) (-5.137, 8.8002) (-5.1588, 8.8132) (-5.1808, 8.8261) (-5.2028, 8.8389) (-5.2249, 8.8516) (-5.2472, 8.8642) (-5.2695, 8.8768) (-5.2919, 8.8892) (-5.3145, 8.9016) (-5.3371, 8.9138) (-5.3598, 8.926) (-5.3826, 8.9381) (-5.4056, 8.9501) (-5.424, 8.9596) (-5.4378, 8.9667) (-5.4471, 8.9714) (-5.4517, 8.9738) knots 0 0 0 0 0 0 0.01428571 0.02857143 0.04285714 0.05714286 0.07142857 0.08571429 0.1 0.11428571 0.12857143 0.14285714 0.15714286 0.17142857 0.18571429 0.2 0.21428571 0.22857143 0.24285714 0.25714286 0.27142857 0.28571429 0.3 0.31428571 0.32857143 0.34285714 0.35714286 0.37142857 0.38571429 0.4 0.41428571 0.42857143 0.44285714 0.45714286 0.47142857 0.48571429 0.5 0.51428571 0.52857143 0.54285714 0.55714286 0.57142857 0.58571429 0.6 0.61428571 0.62857143 0.64285714 0.65714286 0.67142857 0.68571429 0.7 0.71428571 0.72857143 0.74285714 0.75714286 0.77142857 0.78571429 0.8 0.81428571 0.82857143 0.84285714 0.85714286 0.87142857 0.88571429 0.9 0.91428571 0.92857143 0.94285714 0.95714286 0.97142857 0.98571429 1 1 1 1 1 1
  arc A33 (-5.4517, 8.9738) -> (-6.028, 8.5973) centre (0, 0) ccw
  spline S33 degree 5 poles (-6.028, 8.5973) (-6.0277, 8.5921) (-6.0271, 8.5817) (-6.0262, 8.5662) (-6.0249, 8.5455) (-6.0231, 8.5197) (-6.0212, 8.4939) (-6.0192, 8.4682) (-6.017, 8.4426) (-6.0148, 8.417) (-6.0124, 8.3914) (-6.0099, 8.3659) (-6.0072, 8.3405) (-6.0045, 8.3151) (-6.0016, 8.2898) (-5.9986, 8.2645) (-5.9955, 8.2393) (-5.9922, 8.2142) (-5.9889, 8.1891) (-5.9854, 8.1641) (-5.9817, 8.1391) (-5.978, 8.1142) (-5.9741, 8.0894) (-5.9701, 8.0646) (-5.966, 8.0399) (-5.9617, 8.0153) (-5.9573, 7.9907) (-5.9528, 7.9662) (-5.9481, 7.9417) (-5.9433, 7.9174) (-5.9384, 7.8931) (-5.9333, 7.8688) (-5.9282, 7.8447) (-5.9228, 7.8206) (-5.9174, 7.7966) (-5.9118, 7.7727) (-5.906, 7.7488) (-5.9002, 7.7251) (-5.8942, 7.7014) (-5.888, 7.6778) (-5.8817, 7.6542) (-5.8753, 7.6308) (-5.8687, 7.6074) (-5.8619, 7.5842) (-5.8551, 7.561) (-5.848, 7.5379) (-5.8408, 7.5149) (-5.8335, 7.492) (-5.826, 7.4692) (-5.8184, 7.4465) (-5.8106, 7.4239) (-5.8026, 7.4015) (-5.7945, 7.3791) (-5.7861, 7.3568) (-5.7776, 7.3347) (-5.769, 7.3127) (-5.7601, 7.2907) (-5.7511, 7.2689) (-5.742, 7.2472) (-5.7327, 7.2256) (-5.7231, 7.2042) (-5.7133, 7.183) (-5.7032, 7.1619) (-5.6928, 7.141) (-5.6822, 7.1203) (-5.6714, 7.0998) (-5.6605, 7.0793) (-5.6495, 7.059) (-5.6382, 7.0388) (-5.6267, 7.0188) (-5.6145, 6.9993) (-5.6042, 6.9841) (-5.596, 6.973) (-5.5904, 6.9658) (-5.5875, 6.9622) knots -1 -1 -1 -1 -1 -1 -0.98571429 -0.97142857 -0.95714286 -0.94285714 -0.92857143 -0.91428571 -0.9 -0.88571429 -0.87142857 -0.85714286 -0.84285714 -0.82857143 -0.81428571 -0.8 -0.78571429 -0.77142857 -0.75714286 -0.74285714 -0.72857143 -0.71428571 -0.7 -0.68571429 -0.67142857 -0.65714286 -0.64285714 -0.62857143 -0.61428571 -0.6 -0.58571429 -0.57142857 -0.55714286 -0.54285714 -0.52857143 -0.51428571 -0.5 -0.48571429 -0.47142857 -0.45714286 -0.44285714 -0.42857143 -0.41428571 -0.4 -0.38571429 -0.37142857 -0.35714286 -0.34285714 -0.32857143 -0.31428571 -0.3 -0.28571429 -0.27142857 -0.25714286 -0.24285714 -0.22857143 -0.21428571 -0.2 -0.18571429 -0.17142857 -0.15714286 -0.14285714 -0.12857143 -0.11428571 -0.1 -0.08571429 -0.07142857 -0.05714286 -0.04285714 -0.02857143 -0.01428571 0 0 0 0 0 0
  line L33 (-5.5875, 6.9622) -> (-5.164, 6.4329)
  arc A34 (-5.164, 6.4329) -> (-5.9845, 5.6776) centre (0, 0) ccw
  line L34 (-5.9845, 5.6776) -> (-6.477, 6.1434)
  spline S34 degree 5 poles (-6.477, 6.1434) (-6.4804, 6.1465) (-6.4871, 6.1527) (-6.4975, 6.1618) (-6.5118, 6.1733) (-6.5302, 6.1871) (-6.5491, 6.2002) (-6.5683, 6.2131) (-6.5877, 6.2258) (-6.6072, 6.2384) (-6.6268, 6.2508) (-6.6465, 6.2631) (-6.6665, 6.2751) (-6.6866, 6.2869) (-6.707, 6.2985) (-6.7275, 6.3098) (-6.7483, 6.3209) (-6.7692, 6.3318) (-6.7902, 6.3425) (-6.8113, 6.3531) (-6.8325, 6.3636) (-6.8539, 6.3739) (-6.8754, 6.384) (-6.897, 6.394) (-6.9188, 6.4038) (-6.9406, 6.4134) (-6.9626, 6.4229) (-6.9847, 6.4323) (-7.0069, 6.4415) (-7.0293, 6.4505) (-7.0517, 6.4594) (-7.0742, 6.4682) (-7.0968, 6.4769) (-7.1196, 6.4854) (-7.1424, 6.4937) (-7.1653, 6.5019) (-7.1883, 6.51) (-7.2114, 6.518) (-7.2346, 6.5258) (-7.2579, 6.5335) (-7.2813, 6.541) (-7.3048, 6.5484) (-7.3283, 6.5557) (-7.352, 6.5629) (-7.3757, 6.5699) (-7.3995, 6.5768) (-7.4234, 6.5836) (-7.4474, 6.5903) (-7.4714, 6.5968) (-7.4956, 6.6032) (-7.5198, 6.6095) (-7.5441, 6.6157) (-7.5684, 6.6217) (-7.5928, 6.6276) (-7.6174, 6.6334) (-7.6419, 6.6391) (-7.6666, 6.6447) (-7.6913, 6.6501) (-7.7161, 6.6554) (-7.741, 6.6606) (-7.7659, 6.6657) (-7.7909, 6.6706) (-7.8159, 6.6755) (-7.8411, 6.6802) (-7.8663, 6.6848) (-7.8915, 6.6893) (-7.9169, 6.6937) (-7.9422, 6.6979) (-7.9677, 6.702) (-7.9932, 6.7061) (-8.0188, 6.71) (-8.0393, 6.713) (-8.0547, 6.7152) (-8.065, 6.7167) (-8.0701, 6.7174) knots 0 0 0 0 0 0 0.01428571 0.02857143 0.04285714 0.05714286 0.07142857 0.08571429 0.1 0.11428571 0.12857143 0.14285714 0.15714286 0.17142857 0.18571429 0.2 0.21428571 0.22857143 0.24285714 0.25714286 0.27142857 0.28571429 0.3 0.31428571 0.32857143 0.34285714 0.35714286 0.37142857 0.38571429 0.4 0.41428571 0.42857143 0.44285714 0.45714286 0.47142857 0.48571429 0.5 0.51428571 0.52857143 0.54285714 0.55714286 0.57142857 0.58571429 0.6 0.61428571 0.62857143 0.64285714 0.65714286 0.67142857 0.68571429 0.7 0.71428571 0.72857143 0.74285714 0.75714286 0.77142857 0.78571429 0.8 0.81428571 0.82857143 0.84285714 0.85714286 0.87142857 0.88571429 0.9 0.91428571 0.92857143 0.94285714 0.95714286 0.97142857 0.98571429 1 1 1 1 1 1
  arc A35 (-8.0701, 6.7174) -> (-8.4929, 6.1741) centre (0, 0) ccw
  spline S35 degree 5 poles (-8.4929, 6.1741) (-8.491, 6.1693) (-8.487, 6.1597) (-8.4811, 6.1453) (-8.4731, 6.1262) (-8.4631, 6.1024) (-8.4529, 6.0786) (-8.4427, 6.055) (-8.4323, 6.0314) (-8.4218, 6.0079) (-8.4113, 5.9845) (-8.4006, 5.9613) (-8.3899, 5.9381) (-8.3791, 5.9149) (-8.3681, 5.8919) (-8.3571, 5.869) (-8.3459, 5.8462) (-8.3347, 5.8235) (-8.3234, 5.8008) (-8.3119, 5.7783) (-8.3004, 5.7559) (-8.2888, 5.7335) (-8.277, 5.7113) (-8.2652, 5.6892) (-8.2533, 5.6671) (-8.2412, 5.6452) (-8.2291, 5.6234) (-8.2168, 5.6017) (-8.2045, 5.5801) (-8.1921, 5.5586) (-8.1795, 5.5372) (-8.1669, 5.5159) (-8.1541, 5.4948) (-8.1413, 5.4737) (-8.1283, 5.4528) (-8.1152, 5.432) (-8.1021, 5.4113) (-8.0888, 5.3907) (-8.0754, 5.3703) (-8.0619, 5.3499) (-8.0484, 5.3297) (-8.0347, 5.3096) (-8.0208, 5.2897) (-8.0069, 5.2699) (-7.9929, 5.2502) (-7.9787, 5.2307) (-7.9645, 5.2112) (-7.9501, 5.192) (-7.9356, 5.1728) (-7.921, 5.1538) (-7.9063, 5.135) (-7.8915, 5.1163) (-7.8765, 5.0978) (-7.8614, 5.0795) (-7.8461, 5.0613) (-7.8308, 5.0433) (-7.8153, 5.0254) (-7.7997, 5.0077) (-7.784, 4.9901) (-7.7682, 4.9727) (-7.7522, 4.9556) (-7.736, 4.9387) (-7.7196, 4.922) (-7.703, 4.9057) (-7.6863, 4.8895) (-7.6694, 4.8736) (-7.6525, 4.8578) (-7.6354, 4.8421) (-7.6182, 4.8267) (-7.6008, 4.8116) (-7.583, 4.797) (-7.5683, 4.786) (-7.557, 4.7782) (-7.5493, 4.7732) (-7.5454, 4.7707) knots -1 -1 -1 -1 -1 -1 -0.98571429 -0.97142857 -0.95714286 -0.94285714 -0.92857143 -0.91428571 -0.9 -0.88571429 -0.87142857 -0.85714286 -0.84285714 -0.82857143 -0.81428571 -0.8 -0.78571429 -0.77142857 -0.75714286 -0.74285714 -0.72857143 -0.71428571 -0.7 -0.68571429 -0.67142857 -0.65714286 -0.64285714 -0.62857143 -0.61428571 -0.6 -0.58571429 -0.57142857 -0.55714286 -0.54285714 -0.52857143 -0.51428571 -0.5 -0.48571429 -0.47142857 -0.45714286 -0.44285714 -0.42857143 -0.41428571 -0.4 -0.38571429 -0.37142857 -0.35714286 -0.34285714 -0.32857143 -0.31428571 -0.3 -0.28571429 -0.27142857 -0.25714286 -0.24285714 -0.22857143 -0.21428571 -0.2 -0.18571429 -0.17142857 -0.15714286 -0.14285714 -0.12857143 -0.11428571 -0.1 -0.08571429 -0.07142857 -0.05714286 -0.04285714 -0.02857143 -0.01428571 0 0 0 0 0 0
  line L35 (-7.5454, 4.7707) -> (-6.9729, 4.4077)
  arc A36 (-6.9729, 4.4077) -> (-7.5038, 3.4268) centre (0, 0) ccw
  line L36 (-7.5038, 3.4268) -> (-8.1208, 3.7074)
  spline S36 degree 5 poles (-8.1208, 3.7074) (-8.125, 3.7093) (-8.1334, 3.713) (-8.1462, 3.7182) (-8.1634, 3.7245) (-8.1853, 3.7315) (-8.2075, 3.7378) (-8.2298, 3.7437) (-8.2523, 3.7494) (-8.2748, 3.755) (-8.2974, 3.7604) (-8.32, 3.7656) (-8.3428, 3.7705) (-8.3657, 3.7751) (-8.3887, 3.7794) (-8.4118, 3.7835) (-8.435, 3.7872) (-8.4583, 3.7907) (-8.4817, 3.7941) (-8.5051, 3.7973) (-8.5286, 3.8003) (-8.5521, 3.8031) (-8.5757, 3.8057) (-8.5994, 3.8081) (-8.6232, 3.8103) (-8.647, 3.8123) (-8.6709, 3.8142) (-8.6948, 3.8158) (-8.7188, 3.8173) (-8.7429, 3.8186) (-8.767, 3.8198) (-8.7911, 3.8208) (-8.8153, 3.8216) (-8.8396, 3.8222) (-8.8639, 3.8227) (-8.8882, 3.8231) (-8.9126, 3.8232) (-8.9371, 3.8232) (-8.9616, 3.8231) (-8.9861, 3.8228) (-9.0107, 3.8224) (-9.0353, 3.8218) (-9.0599, 3.821) (-9.0846, 3.8201) (-9.1093, 3.8191) (-9.1341, 3.8179) (-9.1589, 3.8165) (-9.1837, 3.815) (-9.2086, 3.8134) (-9.2335, 3.8116) (-9.2584, 3.8097) (-9.2834, 3.8077) (-9.3084, 3.8055) (-9.3334, 3.8031) (-9.3585, 3.8007) (-9.3836, 3.798) (-9.4087, 3.7953) (-9.4338, 3.7924) (-9.459, 3.7894) (-9.4842, 3.7862) (-9.5094, 3.7829) (-9.5347, 3.7795) (-9.56, 3.7759) (-9.5853, 3.7722) (-9.6106, 3.7684) (-9.636, 3.7645) (-9.6613, 3.7604) (-9.6867, 3.7562) (-9.7121, 3.7518) (-9.7376, 3.7473) (-9.763, 3.7427) (-9.7834, 3.7389) (-9.7987, 3.736) (-9.8089, 3.7341) (-9.814, 3.7331) knots 0 0 0 0 0 0 0.01428571 0.02857143 0.04285714 0.05714286 0.07142857 0.08571429 0.1 0.11428571 0.12857143 0.14285714 0.15714286 0.17142857 0.18571429 0.2 0.21428571 0.22857143 0.24285714 0.25714286 0.27142857 0.28571429 0.3 0.31428571 0.32857143 0.34285714 0.35714286 0.37142857 0.38571429 0.4 0.41428571 0.42857143 0.44285714 0.45714286 0.47142857 0.48571429 0.5 0.51428571 0.52857143 0.54285714 0.55714286 0.57142857 0.58571429 0.6 0.61428571 0.62857143 0.64285714 0.65714286 0.67142857 0.68571429 0.7 0.71428571 0.72857143 0.74285714 0.75714286 0.77142857 0.78571429 0.8 0.81428571 0.82857143 0.84285714 0.85714286 0.87142857 0.88571429 0.9 0.91428571 0.92857143 0.94285714 0.95714286 0.97142857 0.98571429 1 1 1 1 1 1
  arc A37 (-9.814, 3.7331) -> (-10.0375, 3.0819) centre (0, 0) ccw
  spline S37 degree 5 poles (-10.0375, 3.0819) (-10.0341, 3.078) (-10.0272, 3.0702) (-10.017, 3.0585) (-10.0032, 3.043) (-9.986, 3.0238) (-9.9686, 3.0046) (-9.9513, 2.9856) (-9.9338, 2.9666) (-9.9163, 2.9478) (-9.8987, 2.9291) (-9.8811, 2.9106) (-9.8634, 2.8921) (-9.8456, 2.8738) (-9.8278, 2.8556) (-9.8099, 2.8375) (-9.792, 2.8195) (-9.774, 2.8017) (-9.7559, 2.7839) (-9.7378, 2.7663) (-9.7196, 2.7489) (-9.7013, 2.7315) (-9.683, 2.7143) (-9.6646, 2.6972) (-9.6462, 2.6802) (-9.6277, 2.6634) (-9.6091, 2.6467) (-9.5905, 2.6302) (-9.5718, 2.6137) (-9.5531, 2.5974) (-9.5343, 2.5813) (-9.5154, 2.5653) (-9.4965, 2.5494) (-9.4775, 2.5337) (-9.4584, 2.5181) (-9.4393, 2.5026) (-9.4201, 2.4873) (-9.4009, 2.4722) (-9.3816, 2.4572) (-9.3622, 2.4423) (-9.3428, 2.4276) (-9.3233, 2.4131) (-9.3038, 2.3987) (-9.2842, 2.3845) (-9.2645, 2.3704) (-9.2448, 2.3566) (-9.225, 2.3428) (-9.2052, 2.3293) (-9.1853, 2.3159) (-9.1653, 2.3026) (-9.1453, 2.2896) (-9.1251, 2.2768) (-9.105, 2.2641) (-9.0847, 2.2517) (-9.0644, 2.2394) (-9.044, 2.2274) (-9.0236, 2.2155) (-9.0031, 2.2038) (-8.9826, 2.1922) (-8.9619, 2.181) (-8.9412, 2.1699) (-8.9204, 2.1592) (-8.8995, 2.1488) (-8.8785, 2.1387) (-8.8575, 2.1289) (-8.8363, 2.1193) (-8.8152, 2.1098) (-8.7939, 2.1005) (-8.7727, 2.0915) (-8.7513, 2.0829) (-8.7297, 2.0749) (-8.7122, 2.0693) (-8.699, 2.0656) (-8.6901, 2.0633) (-8.6856, 2.0622) knots -1 -1 -1 -1 -1 -1 -0.98571429 -0.97142857 -0.95714286 -0.94285714 -0.92857143 -0.91428571 -0.9 -0.88571429 -0.87142857 -0.85714286 -0.84285714 -0.82857143 -0.81428571 -0.8 -0.78571429 -0.77142857 -0.75714286 -0.74285714 -0.72857143 -0.71428571 -0.7 -0.68571429 -0.67142857 -0.65714286 -0.64285714 -0.62857143 -0.61428571 -0.6 -0.58571429 -0.57142857 -0.55714286 -0.54285714 -0.52857143 -0.51428571 -0.5 -0.48571429 -0.47142857 -0.45714286 -0.44285714 -0.42857143 -0.41428571 -0.4 -0.38571429 -0.37142857 -0.35714286 -0.34285714 -0.32857143 -0.31428571 -0.3 -0.28571429 -0.27142857 -0.25714286 -0.24285714 -0.22857143 -0.21428571 -0.2 -0.18571429 -0.17142857 -0.15714286 -0.14285714 -0.12857143 -0.11428571 -0.1 -0.08571429 -0.07142857 -0.05714286 -0.04285714 -0.02857143 -0.01428571 0 0 0 0 0 0
  line L37 (-8.6856, 2.0622) -> (-8.0263, 1.9047)
  circle A38 centre (0, 0) radius 2.5
  circle A39 centre (0, 0) radius 8.249
  dimension "d14" = 16.498
  constraint concentric A0 A39
  measures "d14" diameter of A39
extrude "Extruir3" add sketch "Boceto2 (2)" along normal blind 8 contours A0 A2 A4 A6 A8 A10 A12 A14 A16 A18 A20 A22 A24 A26 A28 A30 A32 A34 A36 A39 in component "Spur Gear (19 teeth)"
sketch "Boceto3 (2)" plane through (0, 0, 14) normal (0, 0, 1) x (-1, 0, 0)
  circle A0 centre (0, 0) radius 2.5
  circle A1 centre (0, 0) radius 8.249
  line L0 (3.25, 3.4) -> (-3.25, 3.4)
  line L1 (-3.25, 3.4) -> (-3.25, 5.6)
  line L2 (-3.25, 5.6) -> (3.25, 5.6)
  line L3 (3.25, 5.6) -> (3.25, 3.4)
  line L4 (0, 3.4) -> (0, -0.3783)
  line L5 (-3.25, -3.4) -> (3.25, -3.4)
  line L6 (3.25, -3.4) -> (3.25, -5.6)
  line L7 (3.25, -5.6) -> (-3.25, -5.6)
  line L8 (-3.25, -5.6) -> (-3.25, -3.4)
  line L9 (0, -3.4) -> (0, 0)
  dimension "d17" = 6.5
  dimension "d18" = 2.2
  dimension "d19" = 3.4
  dimension "d37" = 180
  dimension "d38" = 3.4
  constraint horizontal L0
  constraint vertical L1
  constraint horizontal L2
  constraint vertical L3
  constraint midpoint L0 L4.start
  constraint perpendicular L0 L4
  constraint coincident A0.centre L4
  constraint midpoint L5 L9.start
  constraint coincident A0.centre A1.centre
  constraint equal L3 L6
  constraint equal L0 L7
  constraint perpendicular L7 L8
  constraint perpendicular L5 L8
  constraint perpendicular L5 L6
  constraint perpendicular L5 L9
  measures "d17" distance of L1.end L2.end
  measures "d18" distance of L0.end L1.end
  measures "d19" distance of A0.centre L0
  measures "d37" angle of L4 L9
  measures "d38" distance of L9.start A0.centre
extrude "Extruir4" cut sketch "Boceto3 (2)" against normal blind 7 contours L0 L1 L2 L3 | L5 L6 L7 L8 in component "Spur Gear (19 teeth)"
sketch "Boceto4" plane through (0, 0, 14) normal (0, 0, 1) x (-1, 0, 0)
  line L0 (-3.25, 3.4) -> (-3.25, 5.6)
  line L1 (-3.25, 5.6) -> (3.25, 5.6)
  line L2 (3.25, 5.6) -> (3.25, 3.4)
  line L3 (3.25, 3.4) -> (-3.25, 3.4)
  circle A0 centre (0, 0) radius 2.5
  circle A1 centre (0, 0) radius 8.249
  line L4 (4.0257, 7.2) -> (-4.0257, 7.2)
  circle A2 centre (0, 0) radius 8.249
  line L5 (3.25, -3.4) -> (3.25, -5.6)
  line L6 (3.25, -5.6) -> (-3.25, -5.6)
  line L7 (-3.25, -5.6) -> (-3.25, -3.4)
  line L8 (-3.25, -3.4) -> (3.25, -3.4)
  line L9 (-4.0257, -7.2) -> (4.0257, -7.2)
  dimension "d24" = 1.6
  dimension "d39" = 1.6
  constraint coincident A1 L4.start
  constraint coincident A1 L4.end
  constraint horizontal L4
  constraint coincident A1 L9.start
  constraint coincident A1 L9.end
  constraint parallel L6 L9
  measures "d24" distance of L1 L4
  measures "d39" distance of L6 L9
extrude "Extruir5" cut sketch "Boceto4" against normal blind 7 contours A1 L4 A2 | A1 A2 L9 in component "Spur Gear (19 teeth)"
sketch "Boceto5" plane through (0, -7.2, 0) normal (0, -1, 0) x (1, 0, 0)
  line L0 (4.0257, 14) -> (-4.0257, 14)
  line L1 (-4.0257, 14) -> (-4.0257, 7)
  line L2 (-4.0257, 7) -> (4.0257, 7)
  line L3 (4.0257, 7) -> (4.0257, 14)
  circle A0 centre (0, 10.5) radius 1.6
  dimension "d27" = 3.2
  dimension "d28" = 3.5
  measures "d27" diameter of A0
  measures "d28" distance of L0 A0.centre
extrude "Extruir6" cut sketch "Boceto5" against normal blind 6 contours A0 in component "Spur Gear (19 teeth)"
sketch "Boceto7" plane through (0, 7.2, 0) normal (0, 1, 0) x (-1, 0, 0)
  line L0 (4.0257, 14) -> (-4.0257, 14)
  line L1 (-4.0257, 14) -> (-4.0257, 7)
  line L2 (-4.0257, 7) -> (4.0257, 7)
  line L3 (4.0257, 7) -> (4.0257, 14)
  circle A0 centre (0, 10.5) radius 1.6
  dimension "d40" = 3.2
  dimension "d41" = 3.5
  measures "d40" diameter of A0
  measures "d41" distance of L0 A0.centre
extrude "Extruir8" cut sketch "Boceto7" against normal blind 6 contours A0 in component "Spur Gear (19 teeth)"
sketch "Boceto8" plane through (0, 0, 14) normal (0, 0, 1) x (-1, 0, 0)
  line L0 (4.0257, 7.2) -> (-4.0257, 7.2)
  arc A0 (-4.0257, 7.2) -> (-4.0257, -7.2) centre (0, 0) ccw
  line L1 (-4.0257, -7.2) -> (4.0257, -7.2)
  arc A1 (4.0257, -7.2) -> (4.0257, 7.2) centre (0, 0) ccw
  line L2 (-3.25, 3.4) -> (-3.25, 5.6)
  line L3 (-3.25, 5.6) -> (3.25, 5.6)
  line L4 (3.25, 5.6) -> (3.25, 3.4)
  line L5 (3.25, 3.4) -> (-3.25, 3.4)
  line L6 (3.25, -3.4) -> (3.25, -5.6)
  line L7 (3.25, -5.6) -> (-3.25, -5.6)
  line L8 (-3.25, -5.6) -> (-3.25, -3.4)
  line L9 (-3.25, -3.4) -> (3.25, -3.4)
  circle A2 centre (0, 0) radius 2.5
component "Spur Gear (19 teeth)" placed x (1, 0, 0) y (0, 1, 0) z (0, 0, 1) at (0, 0, 0)
